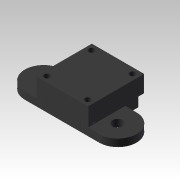
# Autodesk Inventor part: StantonBracket
Saved by Autodesk Inventor 2020 (Build 240168000, 168)
## iProperties
Created: 2022-01-26
Part Number: StantonBracket
Material: Generic
Document SubType Name: Modeling
Designer: DDeGo
Density: 1 g/cm^3
Appearance: Default
Author: DDeGo
Autodesk Inventor part; units mm, degrees
ref_plane "YZ Plane" through (0, 0, 0) normal (1, 0, 0) x (0, 1, 0)
ref_plane "XZ Plane" through (0, 0, 0) normal (0, 1, 0) x (-1, 0, 0)
ref_plane "XY Plane" through (0, 0, 0) normal (0, 0, 1) x (1, 0, 0)
sketch "Sketch1" plane through (0, 0, 0) normal (0, 0, 1) x (1, 0, 0)
  line L0 (-14, -7) -> (14, -7)
  line L1 (14, -7) -> (14, 7)
  line L2 (14, 7) -> (-14, 7)
  line L3 (-14, 7) -> (-14, -7)
  line L4 (-14, -7) -> (14, 7) construction
  line L5 (14, -7) -> (-14, 7) construction
  point P0 (0, 0)
  dimension "d0" = 14
  dimension "d1" = 28
  constraints: 12 end point, 2 midpoint, 2 parallel, 1 horizontal, 1 perpendicular
  measures "d0" distance between parallel lines of L0 L2
  measures "d1" distance of L1.end L2.end
extrude "Extrusion1" add sketch "Sketch1" along normal blind 30
sketch "Sketch2" plane through (-14, -7, 0) normal (0, -1, 0) x (1, 0, 0)
  line L0 (-6, 20) -> (34, 20) construction
  line L1 (28, 30) -> (0, 30) projected
  line L2 (-6, 10) -> (34, 10)
  line L3 (34, 30) -> (-6, 30)
  arc A0 (-6, 30) -> (-6, 10) centre (-6, 20) ccw
  arc A1 (34, 10) -> (34, 30) centre (34, 20) ccw
  line L4 (14, 20) -> (14, 0) construction
  circle A2 centre (-6, 20) radius 3
  circle A3 centre (34, 20) radius 3
  dimension "d4" = 40
  dimension "d5" = 10
  dimension "d8" = 6
  constraints: 10 end point, 4 centre point, 4 point on circle, 4 tangent, 2 coincident, 2 parallel, 1 equal radius, 1 midpoint, 1 point on line, 1 vertical
  measures "d4" distance of L0.start L0.end
  measures "d5" radius of A0
  measures "d8" diameter of A3
extrude "Extrusion2" add sketch "Sketch2" against normal blind 4
sketch "Sketch3" plane through (-14, 7, 0) normal (0, 1, 0) x (1, 0, 0)
  line L0 (28, 0) -> (0, 0) construction
  line L1 (0, 0) -> (0, -30) construction
  line L2 (28, -30) -> (0, -30) construction
  line L3 (28, 0) -> (28, -30) construction
  line L4 (3, -27) -> (3, -3) construction
  line L5 (3, -3) -> (25, -3) construction
  line L6 (25, -3) -> (25, -27) construction
  line L7 (25, -27) -> (3, -27) construction
  circle A0 centre (25, -27) radius 1.75
  circle A1 centre (3, -27) radius 1.75
  circle A2 centre (3, -3) radius 1.75
  circle A3 centre (25, -3) radius 1.75
  point P0 (14, 0)
  dimension "d9" = 22
  dimension "d10" = 24
  dimension "d11" = 3.5
  constraints: 8 end point, 4 centre point, 4 coincident, 3 equal radius, 3 other
  measures "d9" distance of L6.end L4.start
  measures "d10" distance of L5.end L6.end
  measures "d11" diameter of A0
extrude "Extrusion3" cut sketch "Sketch3" against normal through all
sketch "Sketch4" plane through (-14, -7, 0) normal (0, -1, 0) x (1, 0, 0)
  circle A0 centre (25, 27) radius 1.75 projected
  circle A1 centre (25, 27) radius 3
  circle A2 centre (25, 3) radius 1.75 projected
  circle A3 centre (25, 3) radius 3
  circle A4 centre (3, 3) radius 1.75 projected
  circle A5 centre (3, 3) radius 3
  circle A6 centre (3, 27) radius 1.75 projected
  circle A7 centre (3, 27) radius 3
  circle A8 centre (25, 27) radius 1.75 projected
  circle A9 centre (25, 3) radius 1.75 projected
  circle A10 centre (3, 3) radius 1.75 projected
  circle A11 centre (3, 27) radius 1.75 projected
  circle A12 centre (-6, 20) radius 3 projected
  circle A13 centre (34, 20) radius 3 projected
  line L0 (0, 0) -> (0, 10) projected
  line L1 (0, 0) -> (28, 0) projected
  line L2 (28, 0) -> (28, 10) projected
  line L3 (28, 10) -> (34, 10) projected
  arc A14 (34, 10) -> (34, 30) centre (34, 20) ccw projected
  line L4 (34, 30) -> (-6, 30) projected
  arc A15 (-6, 30) -> (-6, 10) centre (-6, 20) ccw projected
  line L5 (-6, 10) -> (0, 10) projected
  point P0 (14, 0)
  point P1 (0, 3)
  point P2 (3, 0)
  point P3 (28, 3)
  point P4 (25, 0)
  dimension "d14" = 6
  constraints: 4 centre point, 4 coincident, 3 equal radius
  measures "d14" diameter of A1
extrude "Extrusion4" cut sketch "Sketch4" against normal blind 5 contours A1 | A7 | A3 | L2 L1 A3 | A5 | A5 L1 L0
body "Solid1"
